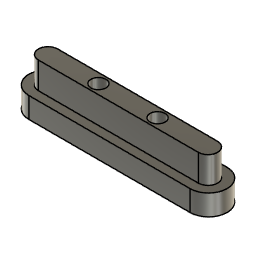
fixated clamp m5 socket head (Autodesk Fusion 360 design; units mm, degrees)
Autodesk Fusion 360 part; units mm, degrees
sketch "Sketch1" plane through (0, 0, 0) normal (0, 0, 1) x (1, 0, 0)
  line L0 (6.25, 0) -> (60.75, 0)
  line L1 (60.75, 12.5) -> (6.25, 12.5)
  arc A0 (6.25, 12.5) -> (0, 6.25) centre (6.25, 6.25) ccw
  arc A1 (0, 6.25) -> (6.25, 0) centre (6.25, 6.25) ccw
  arc A2 (67, 6.25) -> (60.75, 12.5) centre (60.75, 6.25) ccw
  arc A3 (60.75, 0) -> (67, 6.25) centre (60.75, 6.25) ccw
  circle A4 centre (23.5, 6.25) radius 4.3
  circle A5 centre (43.5, 6.25) radius 4.3
  line L2 (33.5, 0) -> (33.5, 12.5) construction
  point P0 (67, 0)
  point P1 (0, 12.5)
  dimension "d1" = 67
  dimension "d2" = 12.5
  dimension "d3" = 6.25
  dimension "d4" = 6.25
  dimension "d5" = 6.25
  dimension "d6" = 6.25
  dimension "d7" = 8.6
  dimension "d8" = 8.6
  dimension "d9" = 20
  dimension "d10" = 10
  constraint horizontal L0
  constraint horizontal L1
  constraint coincident P1 L1
  constraint tangent L1 A0
  constraint coincident origin L0
  constraint tangent L0 A1
  constraint coincident A0.end A1.start
  constraint tangent L1 A2
  constraint coincident P0 L0
  constraint tangent L0 A3
  constraint coincident A2.start A3.end
  constraint midpoint L0 L2.start
  constraint midpoint L1 L2.end
  measures "d1" distance of origin P0
  measures "d2" distance of origin P1
  measures "d3" radius of A0
  measures "d4" radius of A1
  measures "d5" radius of A2
  measures "d6" radius of A3
  measures "d7" diameter of A4
  measures "d8" diameter of A5
  measures "d9" distance of A4.centre A5.centre
  measures "d10" distance of A4.centre L2
extrude "Extrude1" add sketch "Sketch1" against normal blind 5
sketch "Sketch2" plane through (0, 0, -5) normal (0, 0, -1) x (1, 0, 0)
  circle A0 centre (23.5, -6.25) radius 4.3
  circle A1 centre (43.5, -6.25) radius 4.3
  arc A2 (60.75, -12.5) -> (60.75, 0) centre (60.75, -6.25) ccw
  line L0 (60.75, 0) -> (6.25, 0)
  arc A3 (6.25, 0) -> (6.25, -12.5) centre (6.25, -6.25) ccw
  line L1 (6.25, -12.5) -> (60.75, -12.5)
  line L2 (6.45, -9.5) -> (60.55, -9.5)
  line L3 (60.55, -3) -> (6.45, -3)
  line L4 (33.5, 0) -> (33.5, -12.5) construction
  line L5 (0, -6.25) -> (67, -6.25) construction
  line L6 (3.2, -9.5) -> (63.8, -3) construction
  line L7 (3.2, -3) -> (63.8, -9.5) construction
  arc A4 (6.45, -3) -> (3.2, -6.25) centre (6.45, -6.25) ccw
  arc A5 (3.2, -6.25) -> (6.45, -9.5) centre (6.45, -6.25) ccw
  arc A6 (63.8, -6.25) -> (60.55, -3) centre (60.55, -6.25) ccw
  arc A7 (60.55, -9.5) -> (63.8, -6.25) centre (60.55, -6.25) ccw
  circle A8 centre (23.5, -6.25) radius 2.55
  circle A9 centre (43.5, -6.25) radius 2.55
  point P0 (33.5, -6.25)
  point P1 (33.5, -6.25)
  dimension "d13" = 60.6
  dimension "d14" = 6.5
  dimension "d15" = 3.25
  dimension "d16" = 3.25
  dimension "d17" = 3.25
  dimension "d18" = 3.25
  dimension "d19" = 5.1
  dimension "d20" = 5.1
  constraint horizontal L2
  constraint horizontal L3
  constraint midpoint L0 L4.start
  constraint midpoint L1 L4.end
  constraint midpoint A3 L5.start
  constraint midpoint A2 L5.end
  constraint midpoint L7 P1
  constraint midpoint L5 P1
  constraint coincident P1 P0
  constraint coincident L7.start L3
  constraint tangent L3 A4
  constraint coincident L6.start L2
  constraint tangent L2 A5
  constraint coincident A4.end A5.start
  constraint coincident L6.end L3
  constraint tangent L3 A6
  constraint coincident L7.end L2
  constraint tangent L2 A7
  constraint coincident A6.start A7.end
  constraint concentric A0 A8
  constraint concentric A1 A9
  measures "d13" distance of L6.start L7.end
  measures "d14" distance of L6.start L7.start
  measures "d15" radius of A4
  measures "d16" radius of A5
  measures "d17" radius of A6
  measures "d18" radius of A7
  measures "d19" diameter of A8
  measures "d20" diameter of A9
extrude "Extrude2" add sketch "Sketch2" along normal blind 5 contours A0 L2 L3 | A0 A1 L2 L3 | A0 L2 L3 A4 A5 | A1 L2 L3 | A1 L2 L3 A6 A7
extrude "Extrude3" add sketch "Sketch2" along normal blind 1 contours A0 L3 | A0 L2 | A1 L3 | A1 L2 | A2 L0 A3 L1
extrude "Extrude4" add 1 faces at (55.7167, 6.25, -10) along direction (0, 0, -1) blind 1
move_body "Move1" bodies 1 to x (1, 0, 0) y (0, -1, 0) z (0, 0, -1) at (0, 12.5, 0)
extrude "Extrude5" add 1 faces at (42.5167, 1, 6) along direction (0, 0, 1) blind 1
extrude "Extrude6" add 1 faces at (55.7167, 6.25, 11) along direction (0, 0, 1) blind 5
